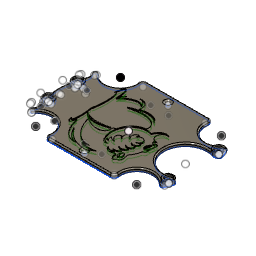
_chassis bottom.d7fee5c5-e527-4b15-a1bc-480d9afafdd5 (Autodesk Fusion 360 design; units mm, degrees)
Autodesk Fusion 360 part; units mm, degrees
sketch "reference" plane through (0, 0, 0) normal (0, 1, 0) x (1, 0, 0)
  line L0 (26.708, 42.6236) -> (27.1586, 42.6236)
  line L1 (-27.225, -55.0823) -> (17.225, -55.0823)
  line L2 (17.225, -55.0823) -> (17.225, -42.3823)
  line L3 (17.225, -42.3823) -> (-27.225, -42.3823)
  line L4 (-27.225, -42.3823) -> (-27.225, -55.0823)
  circle A0 centre (0, 0) radius 65
  line L5 (-27.225, 55.0823) -> (17.225, 55.0823)
  line L6 (17.225, 55.0823) -> (17.225, 42.3823)
  line L7 (17.225, 42.3823) -> (-27.225, 42.3823)
  line L8 (-27.225, 55.0823) -> (-27.225, 42.3823)
  circle A1 centre (0, 0) radius 67.15
  circle A2 centre (68.0978, 18.2467) radius 3
  circle A3 centre (68.0978, 18.2467) radius 1.425
  line L9 (0, 0) -> (82, 0) construction
  line L10 (0, 0) -> (-41, 71.0141) construction
  line L11 (0, 0) -> (-41, -71.0141) construction
  line L12 (87.4769, -0.0257) -> (79.614, 0.0081)
  line L13 (-39.814, 68.9437) -> (-43.7162, 75.77)
  line L14 (-39.8, -68.9518) -> (-43.7607, -75.7444)
  line L15 (0, 0) -> (70.5, 0) construction
  arc A4 (79.614, 0.0081) -> (74.6944, -3.9877) centre (79.5926, -4.9919) ccw
  arc A5 (-39.814, 68.9437) -> (-33.8938, 66.6811) centre (-35.4732, 71.4251) ccw
  arc A6 (-39.8, -68.9518) -> (-40.8007, -62.6934) centre (-44.1194, -66.4332) ccw
  spline S0 degree 5 poles (-33.8938, 66.6811) (-33.483, 66.8179) (-33.0729, 66.9532) (-32.6634, 67.087) (-32.2547, 67.2193) (-31.8466, 67.3502) knots 0.021144 0.021144 0.021144 0.021144 0.021144 0.021144 0.032444 0.032444 0.032444 0.032444 0.032444 0.032444
  line L16 (-32.0549, 67.2834) -> (-31.6382, 67.417)
  spline S1 degree 5 poles (5.0849, 74.3263) (6.6179, 74.3731) (11.2429, 74.4207) (18.7539, 74.0099) (28.746, 72.2391) (40.5731, 67.6689) (52.3904, 59.5578) (62.916, 48.5693) (72.252, 34.9305) (78.8493, 22.0782) (83.3385, 11.4171) (86.1309, 3.8631) (87.4769, -0.0257) knots 0.251095 0.251095 0.251095 0.251095 0.251095 0.251095 0.3 0.4 0.5 0.6 0.7 0.8 0.9 1 1 1 1 1 1
  line L17 (-9.3123, 73.8863) -> (19.482, 74.7663)
  spline S2 degree 5 poles (-40.8007, -62.6934) (-41.1245, -62.4061) (-41.4467, -62.1186) (-41.7673, -61.8309) (-42.0863, -61.543) (-42.4037, -61.255) knots 0.021144 0.021144 0.021144 0.021144 0.021144 0.021144 0.032444 0.032444 0.032444 0.032444 0.032444 0.032444
  line L18 (-42.2416, -61.4021) -> (-42.5658, -61.1079)
  spline S3 degree 5 poles (-66.9109, -32.7595) (-67.718, -31.4553) (-70.0717, -27.4737) (-73.4714, -20.7636) (-76.9339, -11.2248) (-78.8895, 1.3029) (-77.7737, 15.5925) (-73.5202, 30.2022) (-66.3767, 45.1068) (-58.5449, 57.2464) (-51.5568, 66.4647) (-46.4109, 72.66) (-43.7162, 75.77) knots 0.251095 0.251095 0.251095 0.251095 0.251095 0.251095 0.3 0.4 0.5 0.6 0.7 0.8 0.9 1 1 1 1 1 1
  line L19 (-59.9171, -44.0611) -> (-73.9047, -21.4578)
  arc A7 (-66.9109, -32.7595) -> (-37.25, -64.5189) centre (0, 0) ccw
  spline S4 degree 5 poles (74.6944, -3.9877) (74.6075, -4.4118) (74.5196, -4.8346) (74.4308, -5.2561) (74.341, -5.6763) (74.2503, -6.0951) knots 0.021144 0.021144 0.021144 0.021144 0.021144 0.021144 0.032444 0.032444 0.032444 0.032444 0.032444 0.032444
  line L20 (74.2965, -5.8814) -> (74.204, -6.3089)
  spline S5 degree 5 poles (61.826, -41.5668) (61.1001, -42.9178) (58.8287, -46.947) (54.7175, -53.2463) (48.1879, -61.0143) (38.3164, -68.9717) (25.3834, -75.1503) (10.6042, -78.7715) (-5.8753, -80.0373) (-20.3044, -79.3246) (-31.7817, -77.8819) (-39.7199, -76.523) (-43.7607, -75.7444) knots 0.251095 0.251095 0.251095 0.251095 0.251095 0.251095 0.3 0.4 0.5 0.6 0.7 0.8 0.9 1 1 1 1 1 1
  line L21 (68.2252, -29.657) -> (55.4268, -53.4766)
  arc A8 (61.826, -41.5668) -> (74.5, 0) centre (0, 0) ccw
  arc A9 (5.0849, 74.3263) -> (-37.25, 64.5189) centre (0, 0) ccw
  circle A10 centre (18.2467, 68.0978) radius 3
  circle A11 centre (18.2467, 68.0978) radius 1.425
  circle A12 centre (-49.851, 49.851) radius 3
  circle A13 centre (-49.851, 49.851) radius 1.425
  circle A14 centre (-68.0978, -18.2467) radius 3
  circle A15 centre (-68.0978, -18.2467) radius 1.425
  circle A16 centre (-18.2467, -68.0978) radius 3
  circle A17 centre (-18.2467, -68.0978) radius 1.425
  circle A18 centre (49.851, -49.851) radius 3
  circle A19 centre (49.851, -49.851) radius 1.425
  line L22 (0, 0) -> (55.15, 0) construction
  line L23 (0, 0) -> (55.15, 0) construction
  circle A20 centre (42.2474, -35.4497) radius 12
  circle A21 centre (42.2474, 35.4497) radius 12
  line L24 (0, 0) -> (55.15, 0) construction
  line L25 (0, 0) -> (55.15, 0) construction
  circle A22 centre (-42.2474, 35.4497) radius 12
  circle A23 centre (-42.2474, -35.4497) radius 12
  circle A24 centre (0, 0) radius 62.5
  line L26 (-5, -42.3823) -> (-5, 42.3823)
  point P0 (39, 67.55)
  point P1 (-78, 0)
  point P2 (39, -67.55)
  dimension "d9" = 12.7
  dimension "d10" = 44.45
  dimension "d53" = 12.7
  dimension "d54" = 44.45
  dimension "d63" = 130
  dimension "d76" = 134.3
  dimension "d123" = 78
  dimension "d127" = 5
  dimension "d128" = 5
  dimension "d129" = 5
  dimension "d132" = 149
  dimension "d136" = 360
  dimension "d204" = 55.15
  dimension "d206" = 55.15
  dimension "d207" = 24
  dimension "d208" = 24
  dimension "d210" = 55.15
  dimension "d212" = 55.15
  dimension "d213" = 24
  dimension "d214" = 24
  dimension "d227" = 125
  dimension "d232" = 84.7646
  constraint perpendicular L1 L2
  constraint perpendicular L2 L3
  constraint coincident A0.centre A1.centre
  constraint perpendicular L5 L6
  constraint perpendicular L6 L7
  constraint horizontal L9
  constraint horizontal L15
  constraint tangent A4 S4
  constraint tangent L12 A4
  constraint tangent A5 S0
  constraint tangent L13 A5
  constraint tangent A6 S2
  constraint tangent L14 A6
  constraint coincident S0.end A7
  constraint midpoint S0.end L16
  constraint coincident S1.start A7
  constraint midpoint S1.start L17
  constraint coincident L10 A9.end
  constraint coincident S2.end A7
  constraint midpoint S2.end L18
  constraint midpoint S3.start L19
  constraint coincident L11 A7.end
  constraint concentric A7 A8
  constraint coincident S4.end A8
  constraint midpoint S4.end L20
  constraint midpoint S5.start L21
  constraint coincident L9 A8.end
  constraint concentric A8 A9
  constraint horizontal L22
  constraint horizontal L23
  constraint horizontal L24
  constraint horizontal L25
  constraint midpoint L3 L26.start
  constraint midpoint L7 L26.end
  constraint perpendicular L7 L26
  measures "d9" distance of L1.end L2.end
  measures "d10" distance of L2.end L3.end
  measures "d53" distance of L5.end L6.end
  measures "d54" distance of L6.end L7.end
  measures "d63" diameter of A0
  measures "d76" diameter of A1
  measures "d123" distance of A0.centre P0
  measures "d127" radius of A4
  measures "d128" radius of A5
  measures "d129" radius of A6
  measures "d132" diameter of A7
  measures "d204" distance of A0.centre A20.centre
  measures "d206" distance of A0.centre A21.centre
  measures "d207" diameter of A20
  measures "d208" diameter of A21
  measures "d210" distance of A0.centre A23.centre
  measures "d212" distance of A0.centre A22.centre
  measures "d213" diameter of A22
  measures "d214" diameter of A23
  measures "d227" diameter of A24
  measures "d232" distance of L26.start L26.end
sketch "Sketch6" plane through (0, 0, 0) normal (0, 1, 0) x (1, 0, 0)
  line L0 (25.9471, -41.0033) -> (-25.9305, -41.0033)
  arc A0 (53.3928, 17.0259) -> (53.3489, -17.1529) centre (47.6253, -0.0562) ccw
  arc A1 (-28.8946, -37.5404) -> (-53.2717, -27.6825) centre (-42.2338, -35.4569) ccw
  arc A2 (52.1423, -26.2602) -> (28.9106, -37.5367) centre (42.2443, -35.4374) ccw
  arc A3 (55.1761, 27.1684) -> (52.1143, 26.331) centre (54.3168, 24.2941) ccw
  arc A4 (52.1423, -26.2602) -> (55.2056, -27.0935) centre (54.3422, -24.2205) ccw
  arc A5 (58.3345, -19.4651) -> (53.3489, -17.1529) centre (54.6188, -20.946) ccw
  arc A6 (53.3928, 17.0259) -> (58.3852, 19.3275) centre (54.6724, 20.8157) ccw
  circle A7 centre (54.6724, 20.8157) radius 1.425
  circle A8 centre (54.6188, -20.946) radius 1.425
  arc A9 (-56.1762, -2.0025) -> (-56.1762, -2.0026) centre (-0.0106, -0.0004) ccw
  circle A10 centre (-54.8812, 12.3936) radius 1.425
  circle A11 centre (-54.8757, -12.1807) radius 1.425
  arc A12 (28.9662, 37.5373) -> (52.1143, 26.331) centre (42.246, 35.4576) ccw
  line L1 (-54.6751, -2.0026) -> (-54.4366, -2.0026) construction
  line L2 (-49.9389, 12.059) -> (-49.9913, 12.0592)
  circle A13 centre (-46.9939, 12.0456) radius 1.55
  line L3 (-44.9427, 8.8286) -> (-44.9427, 8.8286)
  spline S0 degree 5 poles (-38.2674, -23.601) (-38.2616, -23.5615) (-38.25, -23.4822) (-38.2328, -23.3629) (-38.21, -23.2029) (-38.1818, -23.0019) (-38.1594, -22.8402) (-38.1427, -22.7184) (-38.1316, -22.6368) (-38.1261, -22.596) knots 0 0 0 0 0 0 0.2 0.4 0.6 0.8 1 1 1 1 1 1
  line L4 (-38.2822, -23.7022) -> (-38.2526, -23.4999)
  line L5 (-38.1402, -22.7004) -> (-38.112, -22.4916)
  arc A14 (-53.2884, 27.6676) -> (-28.8973, 37.5386) centre (-42.2488, 35.4595) ccw
  line L6 (-54.333, 19.0252) -> (-54.7513, 17.7702)
  arc A15 (-56.8345, 14.6706) -> (-57.7304, 11.4541) centre (-54.8812, 12.3936) ccw
  spline S1 degree 3 poles (-57.5488, 7.7264) (-57.7948, 6.6323) (-57.9976, 5.5893) (-58.1533, 4.5869) (-58.73, 0.873) (-58.6151, -2.3643) (-57.8493, -6.2568) (-57.7624, -6.6981) (-57.6677, -7.149) (-57.5653, -7.6097) knots 0.254144 0.254144 0.254144 0.254144 0.280571 0.280571 0.280571 0.378481 0.378481 0.378481 0.389582 0.389582 0.389582 0.389582
  arc A16 (-57.7325, -11.2651) -> (-56.8532, -14.4367) centre (-54.8757, -12.1807) ccw
  spline S2 degree 3 poles (-54.8028, -17.5596) (-54.6442, -18.0533) (-54.4816, -18.5512) (-54.3154, -19.0517) knots 0.459488 0.459488 0.459488 0.459488 0.468931 0.468931 0.468931 0.468931
  arc A17 (-55.114, 16.8875) -> (-54.7513, 17.7702) centre (-61.3921, 19.9836) ccw
  arc A18 (-54.333, 19.0252) -> (-55.3983, 25.4709) centre (-60.9739, 21.2385) ccw
  arc A19 (-57.5488, 7.7264) -> (-57.4036, 8.667) centre (-64.3783, 9.2621) ccw
  arc A20 (-57.4291, -8.4753) -> (-57.5653, -7.6097) centre (-64.3985, -9.1286) ccw
  arc A21 (-54.8028, -17.5596) -> (-55.1565, -16.672) centre (-61.4673, -19.7007) ccw
  arc A22 (-55.3823, -25.4886) -> (-54.3154, -19.0517) centre (-60.9588, -21.2575) ccw
  arc A23 (-51.9311, -12.9587) -> (-51.9223, -12.9246) centre (-54.8757, -12.1807) ccw
  line L7 (-53.5111, 9.0025) -> (-53.3775, 9.0028)
  arc A24 (-53.5111, 9.0025) -> (-54.0242, 8.7111) centre (-53.5096, 8.4025) ccw
  line L8 (-25.9331, 41.0003) -> (26.0023, 41.0015)
  arc A25 (-55.4878, -26.5244) -> (-54.9832, -27.5548) centre (-0.0035, 0.0074) ccw
  arc A26 (-54.9996, 27.5386) -> (-55.5043, 26.5064) centre (-0.0035, 0.0074) ccw
  arc A27 (-53.2884, 27.6676) -> (-54.9996, 27.5386) centre (-54.1054, 27.0909) ccw
  arc A28 (-55.5043, 26.5064) -> (-55.3983, 25.4709) centre (-54.6018, 26.0756) ccw
  arc A29 (-54.9832, -27.5548) -> (-53.2717, -27.6825) centre (-54.0893, -27.1066) ccw
  arc A30 (-55.3823, -25.4886) -> (-55.4878, -26.5244) centre (-54.5856, -26.093) ccw
  circle A31 centre (-2, -34.9998) radius 1.425
  circle A32 centre (-1.9946, 35.0003) radius 1.425
  arc A33 (55.2056, -27.0935) -> (58.3345, -19.4651) centre (-0.0035, 0.0074) ccw
  arc A34 (58.3852, 19.3275) -> (55.1761, 27.1684) centre (-0.0035, 0.0074) ccw
  arc A35 (-28.8946, -37.5404) -> (-25.9305, -41.0033) centre (-25.9305, -38.0033) ccw
  arc A36 (25.9471, -41.0033) -> (28.9106, -37.5367) centre (25.9471, -38.0033) ccw
  arc A37 (28.9662, 37.5373) -> (26.0023, 41.0015) centre (26.0024, 38.0015) ccw
  arc A38 (-25.9331, 41.0003) -> (-28.8973, 37.5386) centre (-25.9331, 38.0003) ccw
  circle A39 centre (-54.8812, 12.3936) radius 3
  circle A40 centre (-54.8757, -12.1807) radius 3
  circle A41 centre (-54.8812, 12.3936) radius 4.5
  circle A42 centre (-54.8757, -12.1807) radius 4.5
  arc A43 (51.5521, -17.6527) -> (56.0971, -25.1962) centre (54.6188, -20.946) ccw
  arc A44 (56.1643, 25.0612) -> (51.5973, 17.5303) centre (54.6724, 20.8157) ccw
  arc A45 (57.2747, 22.4063) -> (57.6738, 21.3577) centre (54.6724, 20.8157) ccw
  arc A46 (57.6206, -21.4861) -> (57.2117, -22.552) centre (54.6188, -20.946) ccw
  spline S3 degree 3 poles (25.3331, -1.4893) (25.2569, -1.2607) (25.0664, -0.9273) (24.895, -0.7559) knots 0 0 0 0 1 1 1 1
  spline S4 degree 3 poles (24.895, -0.7559) (24.1997, -0.0415) (23.2948, -0.2891) (22.3042, -1.4798) knots 0 0 0 0 1 1 1 1
  line L9 (22.3042, -1.4798) -> (22.0375, -1.7941)
  line L10 (22.0375, -1.7941) -> (21.7803, -1.556)
  spline S5 degree 3 poles (21.7803, -1.556) (21.6374, -1.4321) (21.4088, -1.2512) (21.2755, -1.1654) knots 0 0 0 0 1 1 1 1
  spline S6 degree 3 poles (21.2755, -1.1654) (21.0373, -1.0226) (20.5516, -0.3653) (20.6278, -0.2987) knots 0 0 0 0 1 1 1 1
  spline S7 degree 3 poles (20.6278, -0.2987) (20.6468, -0.2891) (20.8564, -0.1748) (21.0945, -0.0605) knots 0 0 0 0 1 1 1 1
  spline S8 degree 3 poles (21.0945, -0.0605) (21.5708, 0.1776) (22.7138, 0.9205) (22.7138, 0.9967) knots 0 0 0 0 1 1 1 1
  spline S9 degree 3 poles (22.7138, 0.9967) (22.7138, 1.0253) (22.5137, 1.0348) (22.2661, 1.0158) knots 0 0 0 0 1 1 1 1
  spline S10 degree 3 poles (22.2661, 1.0158) (21.647, 0.9682) (20.6087, 1.2253) (19.942, 1.5778) knots 0 0 0 0 1 1 1 1
  spline S11 degree 3 poles (19.942, 1.5778) (18.9228, 2.1302) (18.0179, 3.2923) (17.7036, 4.4734) knots 0 0 0 0 1 1 1 1
  spline S12 degree 3 poles (17.7036, 4.4734) (17.5322, 5.1115) (17.5417, 6.1593) (17.7131, 6.8546) knots 0 0 0 0 1 1 1 1
  spline S13 degree 3 poles (17.7131, 6.8546) (18.1703, 8.6072) (19.6753, 10.0074) (21.5136, 10.3979) knots 0 0 0 0 1 1 1 1
  spline S14 degree 3 poles (21.5136, 10.3979) (21.9137, 10.4836) (22.3994, 10.5122) (22.7138, 10.4836) knots 0 0 0 0 1 1 1 1
  line L11 (22.7138, 10.4836) -> (23.2376, 10.4265)
  line L12 (23.2376, 10.4265) -> (22.8852, 10.617)
  spline S15 degree 3 poles (22.8852, 10.617) (21.7803, 11.2075) (19.9134, 11.2552) (18.5609, 10.7218) knots 0 0 0 0 1 1 1 1
  spline S16 degree 3 poles (18.5609, 10.7218) (16.694, 9.9979) (15.2747, 8.6644) (14.3889, 6.8165) knots 0 0 0 0 1 1 1 1
  spline S17 degree 3 poles (14.3889, 6.8165) (14.2079, 6.426) (14.0079, 5.8926) (13.9412, 5.6164) knots 0 0 0 0 1 1 1 1
  line L13 (13.9412, 5.6164) -> (13.8269, 5.1115)
  line L14 (13.8269, 5.1115) -> (13.2935, 5.2925)
  spline S18 degree 3 poles (13.2935, 5.2925) (11.579, 5.8831) (8.9692, 6.0736) (7.1309, 5.7307) knots 0 0 0 0 1 1 1 1
  spline S19 degree 3 poles (7.1309, 5.7307) (-0.8225, 4.2638) (-6.0613, -4.3468) (-4.223, -12.9098) knots 0 0 0 0 1 1 1 1
  spline S20 degree 3 poles (-4.223, -12.9098) (-3.8801, -14.5195) (-3.1943, -16.3673) (-2.2322, -18.32) knots 0 0 0 0 1 1 1 1
  spline S21 degree 3 poles (-2.2322, -18.32) (-1.6226, -19.5392) (-0.4034, -20.4345) (0.7681, -20.5107) knots 0 0 0 0 1 1 1 1
  spline S22 degree 3 poles (0.7681, -20.5107) (1.3682, -20.5488) (1.9492, -20.425) (2.1207, -20.2154) knots 0 0 0 0 1 1 1 1
  spline S23 degree 3 poles (2.1207, -20.2154) (2.1969, -20.1297) (2.1112, -20.1011) (1.8159, -20.0916) knots 0 0 0 0 1 1 1 1
  spline S24 degree 3 poles (1.8159, -20.0916) (0.3109, -20.0535) (-1.1845, -18.4724) (-1.4131, -16.7007) knots 0 0 0 0 1 1 1 1
  spline S25 degree 3 poles (-1.4131, -16.7007) (-1.4512, -16.4245) (-1.4417, -16.2435) (-1.3845, -16.2435) knots 0 0 0 0 1 1 1 1
  spline S26 degree 3 poles (-1.3845, -16.2435) (-1.3274, -16.2435) (-1.2893, -16.3007) (-1.2893, -16.3769) knots 0 0 0 0 1 1 1 1
  spline S27 degree 3 poles (-1.2893, -16.3769) (-1.2893, -16.4531) (-1.0702, -16.7483) (-0.813, -17.0436) knots 0 0 0 0 1 1 1 1
  spline S28 degree 3 poles (-0.813, -17.0436) (-0.3368, -17.558) (0.0823, -17.7866) (0.7872, -17.9009) knots 0 0 0 0 1 1 1 1
  spline S29 degree 3 poles (0.7872, -17.9009) (1.111, -17.958) (1.2158, -17.8151) (0.911, -17.7199) knots 0 0 0 0 1 1 1 1
  spline S30 degree 3 poles (0.911, -17.7199) (0.6253, -17.6342) (-0.0415, -16.8531) (-0.2415, -16.3864) knots 0 0 0 0 1 1 1 1
  spline S31 degree 3 poles (-0.2415, -16.3864) (-0.5082, -15.7768) (-0.6416, -14.8719) (-0.5654, -14.2814) knots 0 0 0 0 1 1 1 1
  line L15 (-0.5654, -14.2814) -> (-0.5082, -13.7575)
  line L16 (-0.5082, -13.7575) -> (-0.1844, -14.1385)
  spline S32 degree 3 poles (-0.1844, -14.1385) (0.5967, -15.0529) (1.9778, -15.672) (3.2256, -15.672) knots 0 0 0 0 1 1 1 1
  spline S33 degree 3 poles (3.2256, -15.672) (4.0162, -15.672) (4.3495, -15.5387) (3.7876, -15.4529) knots 0 0 0 0 1 1 1 1
  spline S34 degree 3 poles (3.7876, -15.4529) (2.8255, -15.3005) (1.5016, -14.2718) (1.0063, -13.3098) knots 0 0 0 0 1 1 1 1
  spline S35 degree 3 poles (1.0063, -13.3098) (0.1014, -11.5477) (0.5967, -9.6427) (2.1588, -8.8712) knots 0 0 0 0 1 1 1 1
  line L17 (2.1588, -8.8712) -> (2.6446, -8.6235)
  line L18 (2.6446, -8.6235) -> (2.9494, -9.0807)
  spline S36 degree 3 poles (2.9494, -9.0807) (3.3589, -9.6808) (4.0162, -10.2713) (4.6067, -10.5666) knots 0 0 0 0 1 1 1 1
  spline S37 degree 3 poles (4.6067, -10.5666) (4.8734, -10.7) (5.1116, -10.8143) (5.1496, -10.8143) knots 0 0 0 0 1 1 1 1
  spline S38 degree 3 poles (5.1496, -10.8143) (5.1877, -10.8143) (5.0163, -10.6047) (4.7782, -10.3475) knots 0 0 0 0 1 1 1 1
  spline S39 degree 3 poles (4.7782, -10.3475) (3.178, -8.6426) (3.3208, -5.8898) (5.083, -4.5563) knots 0 0 0 0 1 1 1 1
  spline S40 degree 3 poles (5.083, -4.5563) (5.3021, -4.3849) (5.5402, -4.242) (5.6164, -4.242) knots 0 0 0 0 1 1 1 1
  spline S41 degree 3 poles (5.6164, -4.242) (5.6831, -4.242) (5.7878, -4.442) (5.845, -4.6802) knots 0 0 0 0 1 1 1 1
  spline S42 degree 3 poles (5.845, -4.6802) (6.1879, -6.0422) (7.4357, -7.3472) (8.6644, -7.6329) knots 0 0 0 0 1 1 1 1
  spline S43 degree 3 poles (8.6644, -7.6329) (8.9501, -7.6996) (8.9501, -7.6901) (8.5501, -7.3472) knots 0 0 0 0 1 1 1 1
  spline S44 degree 3 poles (8.5501, -7.3472) (7.3118, -6.2708) (6.8546, -4.3849) (7.4928, -2.9942) knots 0 0 0 0 1 1 1 1
  spline S45 degree 3 poles (7.4928, -2.9942) (8.0072, -1.8798) (8.7501, -1.3845) (9.9122, -1.3845) knots 0 0 0 0 1 1 1 1
  spline S46 degree 3 poles (9.9122, -1.3845) (10.2932, -1.3845) (10.6361, -1.4321) (10.6646, -1.4798) knots 0 0 0 0 1 1 1 1
  spline S47 degree 3 poles (10.6646, -1.4798) (10.6932, -1.5369) (10.6361, -1.7084) (10.5218, -1.8608) knots 0 0 0 0 1 1 1 1
  spline S48 degree 3 poles (10.5218, -1.8608) (10.2646, -2.2227) (9.9503, -3.1085) (9.9503, -3.4514) knots 0 0 0 0 1 1 1 1
  spline S49 degree 3 poles (9.9503, -3.4514) (9.9598, -3.7181) (9.9598, -3.7181) (10.1408, -3.3752) knots 0 0 0 0 1 1 1 1
  spline S50 degree 3 poles (10.1408, -3.3752) (10.5408, -2.6228) (11.5695, -1.956) (12.6649, -1.756) knots 0 0 0 0 1 1 1 1
  spline S51 degree 3 poles (12.6649, -1.756) (13.7126, -1.5655) (14.989, -1.9465) (15.7224, -2.6799) knots 0 0 0 0 1 1 1 1
  spline S52 degree 3 poles (15.7224, -2.6799) (17.2369, -4.2039) (16.4939, -6.6423) (14.2841, -7.3853) knots 0 0 0 0 1 1 1 1
  line L19 (14.2841, -7.3853) -> (13.7126, -7.5758)
  line L20 (13.7126, -7.5758) -> (14.4746, -7.5472)
  spline S53 degree 3 poles (14.4746, -7.5472) (15.2938, -7.4996) (16.0653, -7.2614) (16.6749, -6.8519) knots 0 0 0 0 1 1 1 1
  spline S54 degree 3 poles (16.6749, -6.8519) (17.0845, -6.5756) (17.1321, -6.6137) (17.275, -7.29) knots 0 0 0 0 1 1 1 1
  spline S55 degree 3 poles (17.275, -7.29) (17.456, -8.1187) (17.0368, -9.1474) (16.3034, -9.6808) knots 0 0 0 0 1 1 1 1
  spline S56 degree 3 poles (16.3034, -9.6808) (15.1985, -10.4809) (13.7984, -10.6142) (12.5982, -10.0142) knots 0 0 0 0 1 1 1 1
  spline S57 degree 3 poles (12.5982, -10.0142) (12.341, -9.8999) (12.141, -9.8237) (12.141, -9.8713) knots 0 0 0 0 1 1 1 1
  spline S58 degree 3 poles (12.141, -9.8713) (12.141, -10.0618) (13.2459, -10.919) (13.7412, -11.1095) knots 0 0 0 0 1 1 1 1
  spline S59 degree 3 poles (13.7412, -11.1095) (14.3794, -11.3477) (15.4462, -11.4429) (16.0463, -11.3) knots 0 0 0 0 1 1 1 1
  spline S60 degree 3 poles (16.0463, -11.3) (16.2748, -11.2524) (16.4844, -11.2238) (16.5035, -11.2334) knots 0 0 0 0 1 1 1 1
  spline S61 degree 3 poles (16.5035, -11.2334) (16.6273, -11.3572) (16.6178, -12.0239) (16.4749, -12.4811) knots 0 0 0 0 1 1 1 1
  spline S62 degree 3 poles (16.4749, -12.4811) (15.9796, -14.1956) (13.5126, -15.0529) (11.7886, -14.1004) knots 0 0 0 0 1 1 1 1
  spline S63 degree 3 poles (11.7886, -14.1004) (11.56, -13.9766) (11.379, -13.9099) (11.379, -13.948) knots 0 0 0 0 1 1 1 1
  spline S64 degree 3 poles (11.379, -13.948) (11.379, -14.129) (12.3791, -14.9386) (12.8839, -15.1767) knots 0 0 0 0 1 1 1 1
  spline S65 degree 3 poles (12.8839, -15.1767) (13.3697, -15.4053) (13.5412, -15.4339) (14.4461, -15.4339) knots 0 0 0 0 1 1 1 1
  spline S66 degree 3 poles (14.4461, -15.4339) (15.2081, -15.4339) (15.4748, -15.4625) (15.4748, -15.5577) knots 0 0 0 0 1 1 1 1
  spline S67 degree 3 poles (15.4748, -15.5577) (15.4748, -15.8339) (15.0176, -16.615) (14.608, -17.0246) knots 0 0 0 0 1 1 1 1
  spline S68 degree 3 poles (14.608, -17.0246) (13.4078, -18.2247) (11.4742, -18.4914) (9.8264, -17.6723) knots 0 0 0 0 1 1 1 1
  line L21 (9.8264, -17.6723) -> (9.2835, -17.396)
  line L22 (9.2835, -17.396) -> (9.474, -17.6723)
  spline S69 degree 3 poles (9.474, -17.6723) (10.1693, -18.6438) (11.56, -19.3201) (12.9221, -19.3296) knots 0 0 0 0 1 1 1 1
  spline S70 degree 3 poles (12.9221, -19.3296) (13.3316, -19.3391) (13.665, -19.3487) (13.665, -19.3677) knots 0 0 0 0 1 1 1 1
  spline S71 degree 3 poles (13.665, -19.3677) (13.665, -19.5392) (13.1602, -20.2821) (12.7696, -20.6726) knots 0 0 0 0 1 1 1 1
  spline S72 degree 3 poles (12.7696, -20.6726) (11.8743, -21.5775) (10.5884, -21.9966) (9.2359, -21.8537) knots 0 0 0 0 1 1 1 1
  spline S73 degree 3 poles (9.2359, -21.8537) (8.9215, -21.8156) (8.6548, -21.7966) (8.6358, -21.8156) knots 0 0 0 0 1 1 1 1
  spline S74 degree 3 poles (8.6358, -21.8156) (8.531, -21.9204) (10.0836, -22.5491) (10.5503, -22.5967) knots 0 0 0 0 1 1 1 1
  spline S75 degree 3 poles (10.5503, -22.5967) (11.0837, -22.6538) (11.0932, -22.6538) (10.9313, -22.8348) knots 0 0 0 0 1 1 1 1
  spline S76 degree 3 poles (10.9313, -22.8348) (10.8456, -22.9301) (10.5027, -23.1491) (10.1693, -23.3111) knots 0 0 0 0 1 1 1 1
  spline S77 degree 3 poles (10.1693, -23.3111) (8.5977, -24.0826) (6.5403, -23.6063) (5.2925, -22.1871) knots 0 0 0 0 1 1 1 1
  spline S78 degree 3 poles (5.2925, -22.1871) (4.8258, -21.6537) (4.8258, -21.7871) (5.283, -22.7681) knots 0 0 0 0 1 1 1 1
  spline S79 degree 3 poles (5.283, -22.7681) (5.7878, -23.8635) (6.826, -24.7398) (8.0643, -25.1113) knots 0 0 0 0 1 1 1 1
  spline S80 degree 3 poles (8.0643, -25.1113) (9.0644, -25.4161) (10.3312, -25.3494) (11.2361, -24.9303) knots 0 0 0 0 1 1 1 1
  spline S81 degree 3 poles (11.2361, -24.9303) (11.6076, -24.7589) (12.2267, -24.5398) (12.6172, -24.435) knots 0 0 0 0 1 1 1 1
  spline S82 degree 3 poles (12.6172, -24.435) (13.0078, -24.3398) (13.4173, -24.2255) (13.5221, -24.1969) knots 0 0 0 0 1 1 1 1
  spline S83 degree 3 poles (13.5221, -24.1969) (13.7031, -24.1397) (13.7126, -24.1969) (13.7412, -24.9779) knots 0 0 0 0 1 1 1 1
  spline S84 degree 3 poles (13.7412, -24.9779) (13.8174, -26.921) (14.446, -28.5784) (15.3128, -29.1023) knots 0 0 0 0 1 1 1 1
  spline S85 degree 3 poles (15.3128, -29.1023) (15.6748, -29.3309) (16.3225, -29.3499) (16.7035, -29.1499) knots 0 0 0 0 1 1 1 1
  spline S86 degree 3 poles (16.7035, -29.1499) (17.0464, -28.9784) (17.6083, -28.3212) (17.837, -27.8545) knots 0 0 0 0 1 1 1 1
  spline S87 degree 3 poles (17.837, -27.8545) (17.9989, -27.5021) (17.9989, -27.5021) (18.4847, -27.5497) knots 0 0 0 0 1 1 1 1
  spline S88 degree 3 poles (18.4847, -27.5497) (19.3228, -27.6354) (19.761, -27.2544) (20.0848, -26.159) knots 0 0 0 0 1 1 1 1
  spline S89 degree 3 poles (20.0848, -26.159) (20.4658, -24.8636) (20.3325, -23.0729) (19.7134, -21.2251) knots 0 0 0 0 1 1 1 1
  line L23 (19.7134, -21.2251) -> (19.38, -20.225)
  line L24 (19.38, -20.225) -> (19.7515, -19.7773)
  spline S90 degree 3 poles (19.7515, -19.7773) (20.8183, -18.5009) (21.8946, -16.5293) (22.4661, -14.8148) knots 0 0 0 0 1 1 1 1
  spline S91 degree 3 poles (22.4661, -14.8148) (22.7995, -13.8146) (23.19, -12.1001) (23.19, -11.6334) knots 0 0 0 0 1 1 1 1
  spline S92 degree 3 poles (23.19, -11.6334) (23.19, -11.3953) (23.2186, -11.3858) (23.6662, -11.3858) knots 0 0 0 0 1 1 1 1
  spline S93 degree 3 poles (23.6662, -11.3858) (24.3235, -11.3858) (24.6473, -11.1953) (24.914, -10.6523) knots 0 0 0 0 1 1 1 1
  spline S94 degree 3 poles (24.914, -10.6523) (25.1141, -10.2428) (25.1426, -10.0713) (25.1426, -9.0045) knots 0 0 0 0 1 1 1 1
  spline S95 degree 3 poles (25.1426, -9.0045) (25.1331, -8.0996) (25.0855, -7.6329) (24.9331, -7.0614) knots 0 0 0 0 1 1 1 1
  spline S96 degree 3 poles (24.9331, -7.0614) (24.7426, -6.3661) (24.7331, -6.2804) (24.8664, -6.0232) knots 0 0 0 0 1 1 1 1
  spline S97 degree 3 poles (24.8664, -6.0232) (24.9521, -5.8708) (25.1236, -5.3374) (25.2474, -4.8421) knots 0 0 0 0 1 1 1 1
  spline S98 degree 3 poles (25.2474, -4.8421) (25.5141, -3.7943) (25.5522, -2.1941) (25.3331, -1.4893) knots 0 0 0 0 1 1 1 1
  spline S99 degree 3 poles (25.0474, -4.9564) (24.7045, -6.2994) (23.6567, -7.8139) (22.6661, -8.3949) knots 0 0 0 0 1 1 1 1
  spline S100 degree 3 poles (22.6661, -8.3949) (22.1804, -8.6807) (21.5136, -8.7759) (21.1898, -8.6045) knots 0 0 0 0 1 1 1 1
  spline S101 degree 3 poles (21.1898, -8.6045) (20.5706, -8.2711) (20.3325, -7.4329) (20.5611, -6.328) knots 0 0 0 0 1 1 1 1
  spline S102 degree 3 poles (20.5611, -6.328) (20.9326, -4.5754) (22.3232, -2.7656) (23.5901, -2.4323) knots 0 0 0 0 1 1 1 1
  spline S103 degree 3 poles (23.5901, -2.4323) (24.8188, -2.0989) (25.4855, -3.2514) (25.0474, -4.9564) knots 0 0 0 0 1 1 1 1
  spline S104 degree 3 poles (17.8846, -24.2636) (17.6369, -24.6827) (17.1512, -24.7398) (16.7416, -24.3969) knots 0 0 0 0 1 1 1 1
  spline S105 degree 3 poles (16.7416, -24.3969) (16.1225, -23.8826) (15.5986, -22.3776) (15.7033, -21.4346) knots 0 0 0 0 1 1 1 1
  spline S106 degree 3 poles (15.7033, -21.4346) (15.7415, -21.0632) (15.7319, -20.9965) (15.6462, -21.1394) knots 0 0 0 0 1 1 1 1
  spline S107 degree 3 poles (15.6462, -21.1394) (15.5891, -21.2441) (15.5605, -21.6632) (15.5891, -22.1871) knots 0 0 0 0 1 1 1 1
  spline S108 degree 3 poles (15.5891, -22.1871) (15.6176, -22.911) (15.6748, -23.1587) (15.9129, -23.673) knots 0 0 0 0 1 1 1 1
  spline S109 degree 3 poles (15.9129, -23.673) (16.0748, -24.0159) (16.3511, -24.435) (16.532, -24.6065) knots 0 0 0 0 1 1 1 1
  line L25 (16.532, -24.6065) -> (16.8463, -24.9113)
  line L26 (16.8463, -24.9113) -> (16.5892, -25.1684)
  spline S110 degree 3 poles (16.5892, -25.1684) (16.3034, -25.4542) (15.7891, -25.5209) (15.5224, -25.2923) knots 0 0 0 0 1 1 1 1
  spline S111 degree 3 poles (15.5224, -25.2923) (15.0366, -24.8827) (14.7413, -23.6349) (14.9032, -22.6157) knots 0 0 0 0 1 1 1 1
  spline S112 degree 3 poles (14.9032, -22.6157) (15.0271, -21.7775) (15.2652, -21.2727) (15.8081, -20.7012) knots 0 0 0 0 1 1 1 1
  spline S113 degree 3 poles (15.8081, -20.7012) (16.3701, -20.0916) (16.6082, -20.0916) (17.1797, -20.7012) knots 0 0 0 0 1 1 1 1
  spline S114 degree 3 poles (17.1797, -20.7012) (17.5988, -21.1203) (17.9417, -21.8728) (18.0846, -22.6253) knots 0 0 0 0 1 1 1 1
  spline S115 degree 3 poles (18.0846, -22.6253) (18.1703, -23.092) (18.0656, -23.9588) (17.8846, -24.2636) knots 0 0 0 0 1 1 1 1
  spline S116 degree 3 poles (23.0567, -3.9848) (22.4471, -2.6609) (20.5516, -5.204) (20.7421, -7.0805) knots 0 0 0 0 1 1 1 1
  spline S117 degree 3 poles (20.7421, -7.0805) (20.9516, -9.0807) (23.009, -7.2614) (23.1519, -4.9564) knots 0 0 0 0 1 1 1 1
  spline S118 degree 3 poles (23.1519, -4.9564) (23.1805, -4.4992) (23.1519, -4.1944) (23.0567, -3.9848) knots 0 0 0 0 1 1 1 1
  spline S119 degree 3 poles (8.4834, 9.4454) (8.3024, 10.1788) (7.6547, 11.4457) (7.1213, 12.0934) knots 0 0 0 0 1 1 1 1
  spline S120 degree 3 poles (7.1213, 12.0934) (5.4545, 14.1317) (2.4731, 15.5033) (-1.3845, 16.0082) knots 0 0 0 0 1 1 1 1
  spline S121 degree 3 poles (-1.3845, 16.0082) (-2.9656, 16.2177) (-6.0327, 16.2177) (-7.8139, 16.0082) knots 0 0 0 0 1 1 1 1
  spline S122 degree 3 poles (-7.8139, 16.0082) (-10.1189, 15.7319) (-13.586, 14.9509) (-15.0529, 14.3699) knots 0 0 0 0 1 1 1 1
  spline S123 degree 3 poles (-15.0529, 14.3699) (-15.2624, 14.2937) (-15.3862, 14.2651) (-15.3291, 14.3318) knots 0 0 0 0 1 1 1 1
  spline S124 degree 3 poles (-15.3291, 14.3318) (-15.1577, 14.5032) (-12.2716, 15.7129) (-11.0048, 16.1415) knots 0 0 0 0 1 1 1 1
  spline S125 degree 3 poles (-11.0048, 16.1415) (-3.4609, 18.6752) (3.3971, 18.1227) (6.5498, 14.7127) knots 0 0 0 0 1 1 1 1
  spline S126 degree 3 poles (6.5498, 14.7127) (6.8451, 14.3889) (7.0928, 14.1603) (7.0928, 14.1984) knots 0 0 0 0 1 1 1 1
  spline S127 degree 3 poles (7.0928, 14.1984) (7.0928, 14.227) (6.9594, 14.5222) (6.788, 14.8461) knots 0 0 0 0 1 1 1 1
  spline S128 degree 3 poles (6.788, 14.8461) (6.5879, 15.2176) (6.1784, 15.7319) (5.6259, 16.2844) knots 0 0 0 0 1 1 1 1
  spline S129 degree 3 poles (5.6259, 16.2844) (4.6734, 17.2369) (3.7019, 17.8179) (2.3207, 18.2656) knots 0 0 0 0 1 1 1 1
  spline S130 degree 3 poles (2.3207, 18.2656) (0.4919, 18.8657) (-2.4513, 19.0276) (-4.8611, 18.6752) knots 0 0 0 0 1 1 1 1
  spline S131 degree 3 poles (-4.8611, 18.6752) (-5.8612, 18.5228) (-8.2901, 17.9798) (-8.7283, 17.8084) knots 0 0 0 0 1 1 1 1
  spline S132 degree 3 poles (-8.7283, 17.8084) (-8.8711, 17.7512) (-8.8807, 17.7989) (-8.795, 18.2084) knots 0 0 0 0 1 1 1 1
  spline S133 degree 3 poles (-8.795, 18.2084) (-8.633, 18.98) (-8.6616, 20.9707) (-8.8426, 21.666) knots 0 0 0 0 1 1 1 1
  spline S134 degree 3 poles (-8.8426, 21.666) (-9.3855, 23.7615) (-10.7571, 25.1141) (-12.7383, 25.5332) knots 0 0 0 0 1 1 1 1
  spline S135 degree 3 poles (-12.7383, 25.5332) (-13.5098, 25.7046) (-15.4339, 25.6665) (-15.8625, 25.4855) knots 0 0 0 0 1 1 1 1
  spline S136 degree 3 poles (-15.8625, 25.4855) (-16.0911, 25.3808) (-16.0911, 25.3808) (-15.8149, 25.4284) knots 0 0 0 0 1 1 1 1
  spline S137 degree 3 poles (-15.8149, 25.4284) (-15.2815, 25.5236) (-14.1289, 25.295) (-13.4146, 24.9521) knots 0 0 0 0 1 1 1 1
  spline S138 degree 3 poles (-13.4146, 24.9521) (-12.062, 24.3235) (-10.9571, 22.8947) (-10.5857, 21.3326) knots 0 0 0 0 1 1 1 1
  spline S139 degree 3 poles (-10.5857, 21.3326) (-10.519, 21.0659) (-10.5285, 21.0659) (-11.0238, 21.5327) knots 0 0 0 0 1 1 1 1
  spline S140 degree 3 poles (-11.0238, 21.5327) (-11.6715, 22.1423) (-12.2049, 22.4566) (-13.1002, 22.7233) knots 0 0 0 0 1 1 1 1
  spline S141 degree 3 poles (-13.1002, 22.7233) (-14.0146, 22.9995) (-15.5387, 23.0186) (-16.7197, 22.7709) knots 0 0 0 0 1 1 1 1
  spline S142 degree 3 poles (-16.7197, 22.7709) (-19.7201, 22.1327) (-23.092, 20.0944) (-25.8257, 17.2655) knots 0 0 0 0 1 1 1 1
  line L27 (-25.8257, 17.2655) -> (-26.6924, 16.3701)
  line L28 (-26.6924, 16.3701) -> (-26.7972, 18.1037)
  spline S143 degree 3 poles (-26.7972, 18.1037) (-27.0163, 21.4946) (-27.3497, 23.5043) (-28.0164, 25.5713) knots 0 0 0 0 1 1 1 1
  spline S144 degree 3 poles (-28.0164, 25.5713) (-28.045, 25.6475) (-27.9974, 25.6094) (-27.9212, 25.476) knots 0 0 0 0 1 1 1 1
  spline S145 degree 3 poles (-27.9212, 25.476) (-27.3973, 24.6283) (-26.7877, 21.5708) (-26.5496, 18.5799) knots 0 0 0 0 1 1 1 1
  line L29 (-26.5496, 18.5799) -> (-26.4829, 17.7227)
  line L30 (-26.4829, 17.7227) -> (-25.8638, 18.5799)
  spline S146 degree 3 poles (-25.8638, 18.5799) (-25.1303, 19.5896) (-24.3493, 20.5135) (-23.5492, 21.3041) knots 0 0 0 0 1 1 1 1
  spline S147 degree 3 poles (-23.5492, 21.3041) (-23.1301, 21.7136) (-23.0539, 21.8184) (-23.292, 21.6565) knots 0 0 0 0 1 1 1 1
  spline S148 degree 3 poles (-23.292, 21.6565) (-23.473, 21.5327) (-24.1969, 20.8659) (-24.8827, 20.1706) knots 0 0 0 0 1 1 1 1
  spline S149 degree 3 poles (-24.8827, 20.1706) (-25.578, 19.4753) (-26.1495, 18.9419) (-26.1495, 18.98) knots 0 0 0 0 1 1 1 1
  spline S150 degree 3 poles (-26.1495, 18.98) (-26.1495, 19.1895) (-26.4543, 21.3326) (-26.5781, 22.047) knots 0 0 0 0 1 1 1 1
  spline S151 degree 3 poles (-26.5781, 22.047) (-26.902, 23.7901) (-27.5116, 25.476) (-27.9402, 25.7808) knots 0 0 0 0 1 1 1 1
  spline S152 degree 3 poles (-27.9402, 25.7808) (-28.045, 25.8475) (-28.1879, 26.038) (-28.2736, 26.1904) knots 0 0 0 0 1 1 1 1
  spline S153 degree 3 poles (-28.2736, 26.1904) (-28.5022, 26.6476) (-28.9118, 27) (-29.188, 27) knots 0 0 0 0 1 1 1 1
  spline S154 degree 3 poles (-29.188, 27) (-29.4833, 27) (-29.9404, 26.5714) (-30.1976, 26.0475) knots 0 0 0 0 1 1 1 1
  spline S155 degree 3 poles (-30.1976, 26.0475) (-30.6548, 25.1426) (-31.2263, 22.9805) (-31.4835, 21.1421) knots 0 0 0 0 1 1 1 1
  spline S156 degree 3 poles (-31.4835, 21.1421) (-31.5406, 20.723) (-31.6073, 20.2468) (-31.6454, 20.0944) knots 0 0 0 0 1 1 1 1
  line L31 (-31.6454, 20.0944) -> (-31.6931, 19.8086)
  line L32 (-31.6931, 19.8086) -> (-31.4168, 20.0658)
  spline S157 degree 3 poles (-31.4168, 20.0658) (-30.731, 20.7135) (-30.1405, 20.1515) (-29.6261, 18.3608) knots 0 0 0 0 1 1 1 1
  spline S158 degree 3 poles (-29.6261, 18.3608) (-28.3784, 14.0746) (-28.4736, 4.902) (-29.8166, -0.432) knots 0 0 0 0 1 1 1 1
  spline S159 degree 3 poles (-29.8166, -0.432) (-30.0357, -1.2892) (-30.0357, -1.3654) (-29.9024, -1.9846) knots 0 0 0 0 1 1 1 1
  spline S160 degree 3 poles (-29.9024, -1.9846) (-29.7119, -2.8894) (-29.3309, -5.8327) (-29.188, -7.4329) knots 0 0 0 0 1 1 1 1
  spline S161 degree 3 poles (-29.188, -7.4329) (-29.0356, -9.176) (-29.0356, -13.186) (-29.1785, -14.3385) knots 0 0 0 0 1 1 1 1
  spline S162 degree 3 poles (-29.1785, -14.3385) (-29.3404, -15.5768) (-29.6547, -16.6817) (-29.9309, -17.015) knots 0 0 0 0 1 1 1 1
  spline S163 degree 3 poles (-29.9309, -17.015) (-30.3691, -17.5294) (-30.893, -17.3103) (-31.3502, -16.415) knots 0 0 0 0 1 1 1 1
  spline S164 degree 3 poles (-31.3502, -16.415) (-31.4359, -16.2626) (-31.5121, -16.1483) (-31.5407, -16.1768) knots 0 0 0 0 1 1 1 1
  spline S165 degree 3 poles (-31.5407, -16.1768) (-31.6264, -16.2626) (-31.0073, -18.4724) (-30.712, -19.1105) knots 0 0 0 0 1 1 1 1
  spline S166 degree 3 poles (-30.712, -19.1105) (-29.8071, -21.0632) (-28.7498, -20.2154) (-27.9116, -16.8722) knots 0 0 0 0 1 1 1 1
  spline S167 degree 3 poles (-27.9116, -16.8722) (-27.7783, -16.3578) (-27.6735, -15.853) (-27.6735, -15.7577) knots 0 0 0 0 1 1 1 1
  spline S168 degree 3 poles (-27.6735, -15.7577) (-27.6735, -15.653) (-27.6449, -15.5768) (-27.5973, -15.5768) knots 0 0 0 0 1 1 1 1
  spline S169 degree 3 poles (-27.5973, -15.5768) (-27.5592, -15.5768) (-27.4354, -16.0721) (-27.3116, -16.6817) knots 0 0 0 0 1 1 1 1
  spline S170 degree 3 poles (-27.3116, -16.6817) (-25.8828, -23.8921) (-21.5966, -30.0929) (-16.6912, -32.055) knots 0 0 0 0 1 1 1 1
  spline S171 degree 3 poles (-16.6912, -32.055) (-15.4053, -32.5694) (-14.4338, -32.7503) (-13.0526, -32.7503) knots 0 0 0 0 1 1 1 1
  spline S172 degree 3 poles (-13.0526, -32.7503) (-11.6048, -32.7408) (-10.9667, -32.5979) (-11.9668, -32.5027) knots 0 0 0 0 1 1 1 1
  spline S173 degree 3 poles (-11.9668, -32.5027) (-14.9957, -32.2169) (-18.339, -29.9214) (-20.8631, -26.3876) knots 0 0 0 0 1 1 1 1
  spline S174 degree 3 poles (-20.8631, -26.3876) (-21.587, -25.3685) (-23.1015, -22.7396) (-23.1015, -22.4824) knots 0 0 0 0 1 1 1 1
  spline S175 degree 3 poles (-23.1015, -22.4824) (-23.1015, -22.4443) (-22.8253, -22.8253) (-22.4824, -23.3396) knots 0 0 0 0 1 1 1 1
  spline S176 degree 3 poles (-22.4824, -23.3396) (-20.1678, -26.7972) (-16.7864, -29.75) (-13.1479, -31.493) knots 0 0 0 0 1 1 1 1
  spline S177 degree 3 poles (-13.1479, -31.493) (-10.2332, -32.8837) (-7.5186, -33.4838) (-4.623, -33.3504) knots 0 0 0 0 1 1 1 1
  spline S178 degree 3 poles (-4.623, -33.3504) (-2.4704, -33.2647) (-0.7749, -32.8361) (0.9301, -31.9693) knots 0 0 0 0 1 1 1 1
  spline S179 degree 3 poles (0.9301, -31.9693) (1.7587, -31.5407) (3.4256, -30.4548) (3.3494, -30.3786) knots 0 0 0 0 1 1 1 1
  spline S180 degree 3 poles (3.3494, -30.3786) (3.3304, -30.3596) (2.997, -30.4548) (2.5969, -30.5786) knots 0 0 0 0 1 1 1 1
  spline S181 degree 3 poles (2.5969, -30.5786) (0.9396, -31.1025) (0.0347, -31.2359) (-2.0036, -31.2359) knots 0 0 0 0 1 1 1 1
  spline S182 degree 3 poles (-2.0036, -31.2359) (-4.3468, -31.2454) (-5.5374, -31.0549) (-7.8139, -30.3215) knots 0 0 0 0 1 1 1 1
  line L33 (-7.8139, -30.3215) -> (-8.7664, -30.0071)
  line L34 (-8.7664, -30.0071) -> (-7.5281, -29.95)
  spline S183 degree 3 poles (-7.5281, -29.95) (-6.2899, -29.8928) (-5.5374, -29.75) (-4.4992, -29.369) knots 0 0 0 0 1 1 1 1
  spline S184 degree 3 poles (-4.4992, -29.369) (-4.2039, -29.2642) (-3.9563, -29.1689) (-3.9563, -29.1594) knots 0 0 0 0 1 1 1 1
  spline S185 degree 3 poles (-3.9563, -29.1594) (-3.9563, -29.1499) (-4.5087, -29.1594) (-5.1945, -29.1785) knots 0 0 0 0 1 1 1 1
  spline S186 degree 3 poles (-5.1945, -29.1785) (-6.6995, -29.2261) (-7.671, -29.0927) (-8.995, -28.6641) knots 0 0 0 0 1 1 1 1
  spline S187 degree 3 poles (-8.995, -28.6641) (-14.6719, -26.8067) (-19.9392, -20.8441) (-22.53, -13.3384) knots 0 0 0 0 1 1 1 1
  spline S188 degree 3 poles (-22.53, -13.3384) (-22.9682, -12.062) (-23.4158, -10.4618) (-23.3682, -10.338) knots 0 0 0 0 1 1 1 1
  spline S189 degree 3 poles (-23.3682, -10.338) (-23.3492, -10.2904) (-23.0348, -10.4428) (-22.6729, -10.6809) knots 0 0 0 0 1 1 1 1
  spline S190 degree 3 poles (-22.6729, -10.6809) (-21.6347, -11.3572) (-19.0724, -12.5764) (-17.8056, -12.9955) knots 0 0 0 0 1 1 1 1
  spline S191 degree 3 poles (-17.8056, -12.9955) (-15.8054, -13.6622) (-14.9195, -13.8051) (-12.9098, -13.8146) knots 0 0 0 0 1 1 1 1
  spline S192 degree 3 poles (-12.9098, -13.8146) (-11.3572, -13.8146) (-11.0619, -13.7861) (-10.4047, -13.5956) knots 0 0 0 0 1 1 1 1
  spline S193 degree 3 poles (-10.4047, -13.5956) (-9.2141, -13.2527) (-8.4616, -12.8431) (-7.7663, -12.1478) knots 0 0 0 0 1 1 1 1
  spline S194 degree 3 poles (-7.7663, -12.1478) (-6.6899, -11.081) (-6.2708, -9.9189) (-6.3756, -8.2425) knots 0 0 0 0 1 1 1 1
  spline S195 degree 3 poles (-6.3756, -8.2425) (-6.4042, -7.6901) (-6.4518, -7.1376) (-6.4899, -7.0043) knots 0 0 0 0 1 1 1 1
  spline S196 degree 3 poles (-6.4899, -7.0043) (-6.5375, -6.7661) (-6.4994, -6.7376) (-5.4326, -6.3375) knots 0 0 0 0 1 1 1 1
  spline S197 degree 3 poles (-5.4326, -6.3375) (-4.4897, -5.9756) (-4.3182, -5.8803) (-4.2801, -5.6707) knots 0 0 0 0 1 1 1 1
  spline S198 degree 3 poles (-4.2801, -5.6707) (-2.918, 0.7205) (1.8445, 5.4735) (7.6738, 6.2545) knots 0 0 0 0 1 1 1 1
  line L35 (7.6738, 6.2545) -> (8.5025, 6.3593)
  line L36 (8.5025, 6.3593) -> (8.5596, 6.7879)
  spline S199 degree 3 poles (8.5596, 6.7879) (8.6549, 7.4737) (8.6072, 8.912) (8.4834, 9.4454) knots 0 0 0 0 1 1 1 1
  spline S200 degree 3 poles (-8.814, -7.652) (-17.3294, -10.8714) (-25.1303, -10.3094) (-28.1879, -6.2422) knots 0 0 0 0 1 1 1 1
  spline S201 degree 3 poles (-28.1879, -6.2422) (-28.4355, -5.9089) (-28.6165, -5.6231) (-28.5879, -5.6041) knots 0 0 0 0 1 1 1 1
  spline S202 degree 3 poles (-28.5879, -5.6041) (-28.5689, -5.585) (-28.2736, -5.7851) (-27.9402, -6.0517) knots 0 0 0 0 1 1 1 1
  spline S203 degree 3 poles (-27.9402, -6.0517) (-27.2258, -6.6328) (-25.5685, -7.4614) (-24.3874, -7.852) knots 0 0 0 0 1 1 1 1
  spline S204 degree 3 poles (-24.3874, -7.852) (-20.625, -9.0617) (-15.7101, -9.0998) (-10.6619, -7.9472) knots 0 0 0 0 1 1 1 1
  spline S205 degree 3 poles (-10.6619, -7.9472) (-9.9856, -7.7948) (-9.0807, -7.5662) (-8.6616, -7.4329) knots 0 0 0 0 1 1 1 1
  spline S206 degree 3 poles (-8.6616, -7.4329) (-7.9377, -7.2043) (-7.6901, -7.1471) (-7.7758, -7.2329) knots 0 0 0 0 1 1 1 1
  spline S207 degree 3 poles (-7.7758, -7.2329) (-7.7948, -7.2519) (-8.2616, -7.4424) (-8.814, -7.652) knots 0 0 0 0 1 1 1 1
  point P0 (42.2474, 35.4497)
  point P1 (42.2474, -35.4497)
  point P2 (-42.2474, -35.4497)
  point P3 (-42.2474, 35.4497)
  point P4 (-42.2473, -35.4497)
  point P5 (-42.2474, 35.4497)
  point P6 (42.2443, -35.4374)
  point P7 (42.246, 35.4576)
  point P8 (-9.4894, 28.0017)
  point P9 (5.5003, 28.0002)
  point P10 (-9.5, -28)
  point P11 (5.5279, -27.9998)
  point P12 (-46.9939, 12.0456)
  dimension "d325" = 3
  dimension "d330" = 4
  dimension "d381" = 2.85
  dimension "d382" = 2.85
  dimension "d385" = 6
  dimension "d386" = 6
  dimension "d387" = 2.85
  dimension "d388" = 2.85
  dimension "d610" = 3.1
  dimension "d791" = 7
  dimension "d794" = 7
  dimension "d795" = 7
  dimension "d797" = 7
  dimension "d800" = 7
  dimension "d801" = 7
  dimension "d812" = 0.6
  dimension "d887" = 1
  dimension "d888" = 1
  dimension "d957" = 2.85
  dimension "d959" = 2.85
  dimension "d968" = 3
  dimension "d969" = 3
  dimension "d970" = 3
  dimension "d971" = 3
  dimension "d974" = 9
  dimension "d975" = 9
  dimension "d976" = 9
  dimension "d977" = 9
  dimension "d980" = 6.1
  dimension "d981" = 6.1
  constraint horizontal L0
  constraint tangent A3 A12
  constraint tangent A2 A4
  constraint equal A3 A4
  constraint tangent A0 A5
  constraint tangent A0 A6
  constraint equal A5 A6
  constraint concentric A6 A7
  constraint concentric A5 A8
  constraint concentric A10 A15
  constraint concentric A11 A16
  constraint horizontal L1
  constraint coincident P5 P3
  constraint coincident P6 A2.centre
  constraint coincident P7 A12.centre
  constraint coincident P12 A13.centre
  constraint coincident L2 P12
  constraint coincident A1 S0.end
  constraint midpoint S0.start L4
  constraint midpoint S0.end L5
  constraint concentric A16 A23
  constraint tangent L6 A17
  constraint tangent A15 A17
  constraint tangent L6 A18
  constraint tangent A15 A19
  constraint tangent S1 A19
  constraint tangent S1 A20
  constraint tangent A16 A20
  constraint tangent A16 A21
  constraint tangent S2 A21
  constraint tangent S2 A22
  constraint tangent L7 A24
  constraint tangent A14 A27
  constraint tangent A26 A27
  constraint tangent A18 A28
  constraint tangent A26 A28
  constraint tangent A1 A29
  constraint tangent A25 A29
  constraint tangent A25 A30
  constraint tangent A22 A30
  constraint equal A29 A30
  constraint concentric A33 A34
  constraint tangent L0 A35
  constraint tangent A1 A35
  constraint tangent L0 A36
  constraint tangent A2 A36
  constraint tangent L8 A37
  constraint tangent A12 A37
  constraint tangent L8 A38
  constraint tangent A14 A38
  constraint concentric A15 A39
  constraint concentric A23 A40
  constraint concentric A15 A41
  constraint concentric A40 A42
  constraint concentric A7 A44
  constraint coincident A33 A43.end
  constraint coincident A0 A43.start
  constraint coincident A0 A44.end
  constraint coincident A34 A44.start
  constraint concentric A43 A46
  constraint concentric A6 A45
  constraint coincident A34 A45.end
  constraint coincident A34 A45.start
  constraint coincident A33 A46.end
  constraint coincident A33 A46.start
  constraint coincident A42 A21.end
  constraint coincident A42 A20.start
  constraint coincident A41 A19.end
  constraint coincident A41 A17.start
  measures "d325" radius of A3
  measures "d330" radius of A5
  measures "d381" diameter of A7
  measures "d382" diameter of A8
  measures "d385" diameter of A15
  measures "d386" diameter of A16
  measures "d387" diameter of A10
  measures "d388" diameter of A11
  measures "d610" diameter of A13
  measures "d791" radius of A17
  measures "d794" radius of A18
  measures "d795" radius of A19
  measures "d797" radius of A20
  measures "d800" radius of A21
  measures "d801" radius of A22
  measures "d812" radius of A24
  measures "d887" radius of A28
  measures "d888" radius of A29
  measures "d957" diameter of A31
  measures "d959" diameter of A32
  measures "d968" radius of A35
  measures "d969" radius of A36
  measures "d970" radius of A37
  measures "d971" radius of A38
  measures "d974" diameter of A41
  measures "d975" diameter of A42
  measures "d976" diameter of A43
  measures "d977" diameter of A44
  measures "d980" diameter of A46
  measures "d981" diameter of A45
extrude "Extrude154" add sketch "Sketch6" along normal blind 4 contours A0 A5 A9 A43 A46 | A9 A33 A43 A46 | A9 A16 A40 A42 | A9 A40 A42 | A5 A9 A33 A46 | A0 A6 A9 A44 A45 | A9 A34 A44 A45 | A9 A15 A39 A41 | A9 A39 A41 | A6 A9 A34 A45 makes body 1 at (-50.3813, 1.3333, 12.405) makes body 2 at (57.7126, 2.6667, -21.0597) makes body 3 at (-50.3868, 1.3333, -12.1693) makes body 4 at (57.0413, 2.6667, 22.7991)
fillet "Fillet164" radius 0.5 2 edges at (-57.6727, 4, 11.0959) (-57.6782, 4, -13.4784) on bodies 1 3
fillet "Fillet174" radius 1 2 edges at (-59.0712, 4, 13.808) (-59.0767, 4, -10.7663) on bodies 1 3
extrude "Extrude155" add sketch "Sketch6" along normal blind 2.5 contours L0 A0 A1 A2 A9 A12 A14 L8 A35 A36 A37 A38 A41 A42 A43 A44 | A2 A4 A9 A33 A43 | A1 A9 S2 A21 A22 A25 A29 A30 A42 | A9 A46 | A9 A33 A46 | A9 A11 A16 A40 | A9 A11 A40 | A9 S1 A19 A20 A41 A42 | A3 A9 A12 A34 A44 | A9 A34 A45 | A9 A45 | A9 A10 A15 A39 | A9 A10 A39 | A9 A14 L6 A17 A18 A26 A27 A28 A41 | A13 | S99 S100 S101 S102 S103 | S104 S105 S106 S107 S108 S109 L25 L26 S110 S111 S112 S113 S114 S115 | S200 S201 S202 S203 S204 S205 S206 S207 bodies 1 2 3 4 makes body 5 at (23.9794, 0, 3.0539) makes body 6 at (16.2544, 0, 20.6851) makes body 7 at (-10.3905, 0.8333, 8.2078)
extrude "Extrude156" add sketch "Sketch6" along normal blind 1.75 contours S3 S4 L9 L10 S5 S6 S7 S8 S9 S10 S11 S12 S13 S14 L11 L12 S15 S16 S17 L13 L14 S18 S19 S20 S21 S22 S23 S24 S25 S26 S27 S28 S29 S30 S31 L15 L16 S32 S33 S34 S35 L17 L18 S36 S37 S38 S39 S40 S41 S42 S43 S44 S45 S46 S47 S48 S49 S50 S51 S52 L19 L20 S53 S54 S55 S56 S57 S58 S59 S60 S61 S62 S63 S64 S65 S66 S67 S68 L21 L22 S69 S70 S71 S72 S73 S74 S75 S76 S77 S78 S79 S80 S81 S82 S83 S84 S85 S86 S87 S88 S89 L23 L24 S90 S91 S92 S93 S94 S95 S96 S97 S98 | S116 S117 S118 | S119 S120 S121 S122 S123 S124 S125 S126 S127 S128 S129 S130 S131 S132 S133 S134 S135 S136 S137 S138 S139 S140 S141 S142 L27 L28 S143 S144 S145 L29 L30 S146 S147 S148 S149 S150 S151 S152 S153 S154 S155 S156 L31 L32 S157 S158 S159 S160 S161 S162 S163 S164 S165 S166 S167 S168 S169 S170 S171 S172 S173 S174 S175 S176 S177 S178 S179 S180 S181 S182 L33 L34 S183 S184 S185 S186 S187 S188 S189 S190 S191 S192 S193 S194 S195 S196 S197 S198 L35 L36 S199 bodies 1 5 6 7
fillet "Fillet176" radius 1 28 edges at (53.5254, 2.5, -27.1878) (36.389, 2.5, -23.3591) (28.2819, 2.5, -39.9518) (0.0346, 2.5, -41.0009) (-28.2118, 2.5, -39.9515) (-37.1797, 2.5, -22.9339) (-54.1805, 2.5, -28.0881) (-55.2543, 2.5, -27.0237) (-55.5967, 2.5, -25.9738) (-54.0676, 2.5, -22.38) (-54.5422, 2.5, -18.3977) (-54.9176, 2.5, -17.3227) (-54.9645, 2.5, 17.1097) (-54.562, 2.5, 18.3031) (-54.053, 2.5, 22.4021) (-55.5805, 2.5, 25.9917) (-55.2379, 2.5, 27.0408) (-54.1637, 2.5, 28.1039) (-37.1724, 2.5, 22.9406) (-28.2097, 2.5, 39.9541) (0.0083, 2.5, 41.0033) (28.2275, 2.5, 39.9527) (36.3501, 2.5, 23.2945) (53.5547, 2.5, 27.1153) (-57.4602, 2.5, -8.1942) (-58.517, 2.5, -0.0574) (-57.4836, 2.5, 8.0404) (29.5959, 2.5, 0.033) on bodies 1
chamfer "Chamfer12" distance 1.75 angle 45 2 edges at (-3.3232, 2.5, -35.5156) (-3.3286, 2.5, 34.4845) on bodies 1
